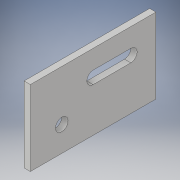
# Autodesk Inventor part: 8.2
Saved by Autodesk Inventor 2017.3 (Build 213256000, 256)
## iProperties
Created: 2017-05-02
Part Number: 8.2
Material: Generic
Document SubType Name: Modeling
Designer: rbibb
Density: 1 g/cm^3
Appearance: Default
Author: rbibb
Autodesk Inventor part; units mm, degrees
ref_plane "YZ Plane" through (0, 0, 0) normal (1, 0, 0) x (0, 1, 0)
ref_plane "XZ Plane" through (0, 0, 0) normal (0, 1, 0) x (-1, 0, 0)
ref_plane "XY Plane" through (0, 0, 0) normal (0, 0, 1) x (1, 0, 0)
sketch "Sketch1" plane through (0, 0, 0) normal (1, 0, 0) x (0, 1, 0)
  line L0 (42.6763, 41.7539) -> (-33.5237, 41.7539)
  line L1 (-33.5237, 41.7539) -> (-33.5237, -85.2461)
  line L2 (-33.5237, -85.2461) -> (42.6763, -85.2461)
  line L3 (42.6763, -85.2461) -> (42.6763, 41.7539)
  point P0 (0, 0)
  dimension "d0" = 76.2
  dimension "d1" = 127
  constraints: 8 end point, 2 parallel, 1 horizontal, 1 perpendicular
  measures "d0" distance of L1.end L2.end
  measures "d1" distance of L2.end L0.start
extrude "Extrusion1" add sketch "Sketch1" along normal blind 6.35
sketch "Sketch3" plane through (6.35, 0, 0) normal (1, 0, 0) x (0, 0, -1)
  arc A0 (59.8461, 10.9263) -> (59.8461, 23.6263) centre (59.8461, 17.2763) ccw
  arc A1 (21.7461, 23.6263) -> (21.7461, 10.9263) centre (21.7461, 17.2763) ccw
  line L0 (21.7461, 23.6263) -> (59.8461, 23.6263)
  line L1 (59.8461, 10.9263) -> (21.7461, 10.9263)
  line L2 (-41.7539, 42.6763) -> (-41.7539, -33.5237) projected
  line L3 (85.2461, 42.6763) -> (-41.7539, 42.6763) projected
  point P0 (0, 0)
  dimension "d4" = 38.1
  dimension "d5" = 101.6
  dimension "d6" = 25.4
  dimension "d7" = 25.4
  dimension "d9" = 6.35
  constraints: 4 end point, 4 point on circle, 3 tangent, 2 centre point, 1 equal radius
  measures "d4" distance of A0.centre A1.centre
  measures "d5" distance from line of A0.centre L2
  measures "d6" distance from line of A1.centre L3
  measures "d7" distance from line of L3 A0.centre
  measures "d9" radius of A0
extrude "Extrusion2" cut sketch "Sketch3" against normal blind 6.35
sketch "Sketch4" plane through (6.35, 0, 0) normal (1, 0, 0) x (0, 0, -1)
  circle A0 centre (-10.0039, -8.1237) radius 6.35
  line L0 (-41.7539, 42.6763) -> (-41.7539, -33.5237) projected
  line L1 (85.2461, 42.6763) -> (-41.7539, 42.6763) projected
  point P0 (0, 0)
  dimension "d12" = 31.75
  dimension "d13" = 50.8
  dimension "d14" = 12.7
  constraints: 1 centre point
  measures "d12" distance from line of L0 A0.centre
  measures "d13" distance from line of L1 A0.centre
  measures "d14" diameter of A0
extrude "Extrusion3" cut sketch "Sketch4" against normal blind 6.35
equation "\"d1\" = 1.66667 * d0"
equation "\"d2\" = 0.05 * d1"
equation "\"d4\" = 0.5 * d0"
equation "\"d5\" = 0.8 * d1"
equation "\"d6\" = 0.333333 * d0"
equation "\"d7\" = 0.333333 * d0"
equation "\"d9\" = d2"
equation "\"d10\" = 0.05 * d1"
equation "\"d12\" = 0.25 * d1"
equation "\"d13\" = 0.666667 * d0"
equation "\"d15\" = 0.05 * d1"
body "Solid1"
